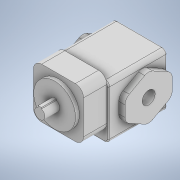
# Autodesk Inventor part: Motor Pump
Saved by Autodesk Inventor 2020 (Build 240168000, 168)
## iProperties
Created: 2020-10-14
Part Number: Motor Pump
Material: Generic
Document SubType Name: Modeling
Designer: jtri402
Density: 1 g/cm^3
Appearance: Default
Author: jtri402
Autodesk Inventor part; units mm, degrees
ref_plane "YZ Plane" through (0, 0, 0) normal (1, 0, 0) x (0, 1, 0)
sketch "Sketch1" plane through (0, 0, 0) normal (0, 0, 1) x (1, 0, 0)
  line L0 (-65, 65) -> (65, 65)
  line L1 (65, 65) -> (65, -65)
  line L2 (65, -65) -> (-65, -65)
  line L3 (-65, -65) -> (-65, 65)
  point P0 (0, 0)
  dimension "d0" = 130
  dimension "d1" = 130
  dimension "d2" = 65
  dimension "d3" = 65
  constraints: 8 end point, 2 parallel, 1 horizontal, 1 perpendicular
  measures "d0" distance of L0.start L0.end
  measures "d1" distance of L0.end L1.end
  measures "d2" distance from line of point (0, 0) L0
  measures "d3" distance from line of L1 point (0, 0)
extrude "Extrusion1" add sketch "Sketch1" along normal blind 203.2
ref_plane "Work Plane2" through (65, -55, 2) normal (1, 0, 0) x (0, 0, -1)
sketch "Sketch2" plane through (65, -55, 2) normal (1, 0, 0) x (0, 0, -1)
  line L0 (0, 110) -> (0, 0) projected
  line L1 (-115, 80) -> (0, 80)
  line L2 (0, 80) -> (0, 30)
  line L3 (0, 30) -> (-115, 30)
  line L4 (-115, 30) -> (-115, 80)
  line L5 (-201.2, -10) -> (2, -10) projected
  line L6 (2, 120) -> (-201.2, 120) projected
  line L7 (-57.5, 111.6) -> (-115, 80)
  line L8 (-57.5, 111.6) -> (0, 80)
  line L9 (-57.5, -1.6) -> (-115, 30)
  line L10 (-57.5, -1.6) -> (0, 30)
  point P0 (2, 55)
  point P1 (-199.2, -10)
  point P2 (0, -10)
  point P3 (0, 120)
  point P4 (-199.2, 120)
  point P5 (0, 80)
  dimension "d8" = 50
  dimension "d9" = 115
  dimension "d10" = 130
  dimension "d11" = 40
  constraints: 16 end point, 4 parallel, 1 horizontal, 1 perpendicular, 1 point on line
  measures "d8" distance of L3.end L1.start
  measures "d9" distance of L1.start L1.end
  measures "d10" distance between parallel lines of L5 L6
  measures "d11" distance between parallel lines of L1 L6
extrude "Extrusion2" add sketch "Sketch2" along normal blind 15
sketch "Sketch3" plane through (80, -55, 2) normal (1, 0, 0) x (0, 0, -1)
  circle A0 centre (-57.5, 55) radius 15.8
  point P0 (2, 55)
  dimension "d18" = 31.6
  constraints: 1 centre point
  measures "d18" diameter of A0
ref_plane "Work Plane1" through (-65, -55, 2) normal (-1, 0, 0) x (0, 0, 1)
sketch "Sketch4" plane through (-65, -55, 2) normal (-1, 0, 0) x (0, 0, 1)
  line L0 (0, 110) -> (0, 68.1701) projected
  line L1 (0, 80) -> (115.3, 80)
  line L2 (115.3, 80) -> (115.3, 30)
  line L3 (115.3, 30) -> (0, 30)
  line L4 (0, 30) -> (0, 80)
  line L5 (201.2, 120) -> (-2, 120) projected
  line L6 (-2, -10) -> (201.2, -10) projected
  line L7 (0, 80) -> (57.5, 110.755)
  arc A0 (60.3849, 110.0145) -> (54.6151, 110.0145) centre (57.5, 104.765) ccw projected
  line L8 (60.3849, 110.0145) -> (104.6325, 85.6976) projected
  line L9 (57.5, 110.755) -> (115.3, 80)
  line L10 (115.3, 30) -> (57.8, -0.755)
  line L11 (57.8, -0.755) -> (0, 30)
  point P0 (-2, 55)
  point P1 (199.2, 120)
  point P2 (0, 120)
  point P3 (0, -10)
  point P4 (199.2, -10)
  dimension "d19" = 115.3
  dimension "d20" = 50
  dimension "d21" = 40
  dimension "d22" = 130
  constraints: 16 end point, 4 parallel, 1 horizontal, 1 perpendicular, 1 point on circle, 1 point on line
  measures "d19" distance of L1.start L1.end
  measures "d20" distance of L3.end L1.start
  measures "d21" distance between parallel lines of L1 L5
  measures "d22" distance between parallel lines of L6 L5
extrude "Extrusion3" add sketch "Sketch4" along normal blind 15
extrude "Extrusion4" cut sketch "Sketch3" against normal blind 160
sketch "Sketch6" plane through (0, 0, 203.2) normal (0, 0, 1) x (1, 0, 0)
  line L0 (-65, 65) -> (-65, -65) projected
  line L1 (65, -65) -> (65, 65) projected
  line L2 (-65, 65) -> (65, 65)
  line L3 (65, 65) -> (65, -65)
  line L4 (65, -65) -> (-65, -65)
  line L5 (-65, -65) -> (-65, 65)
  point P0 (0, 0)
  constraints: 8 end point, 2 parallel, 1 horizontal, 1 perpendicular
extrude "Extrusion5" cut sketch "Sketch6" against normal blind 60.9
fillet "Fillet8" radius 3 8 edges at (0, 65, 142.3) (65, 0, 142.3) (0, -65, 142.3) (-65, 0, 142.3) (65, 0, 0) (0, 65, 0) (-65, 0, 0) (0, -65, 0)
fillet "Fillet8" radius 10 4 edges at (65, 65, 71.15) (-65, 65, 71.15) (-65, -65, 71.15) (65, -65, 71.15)
fillet "Fillet8" radius 20 12 edges at (72.5, 56.6, 59.5) (72.5, 25, 117) (72.5, -25, 117) (72.5, -25, 2) (72.5, 25, 2) (72.5, -56.6, 59.5) (-72.5, -55.755, 59.8) (-72.5, -25, 2) (-72.5, 25, 2) (-72.5, 55.755, 59.5) (-72.5, 25, 117.3) (-72.5, -25, 117.3)
sketch "Sketch7" plane through (0, 0, 142.3) normal (0, 0, 1) x (1, 0, 0)
  line L0 (-61, 79.5) -> (61, 79.5)
  line L1 (61, 79.5) -> (61, -42.5)
  line L2 (61, -42.5) -> (-61, -42.5)
  line L3 (-61, -42.5) -> (-61, 79.5)
  line L4 (-65, 55) -> (-65, -55) projected
  line L5 (-55, -65) -> (55, -65) projected
  point P0 (0, 0)
  dimension "d38" = 122
  dimension "d39" = 122
  dimension "d40" = 4
  dimension "d41" = 22.5
  constraints: 8 end point, 2 parallel, 1 horizontal, 1 perpendicular
  measures "d38" distance of L0.start L0.end
  measures "d39" distance of L0.end L1.end
  measures "d40" distance between parallel lines of L3 L4
  measures "d41" distance between parallel lines of L5 L2
extrude "Extrusion6" add sketch "Sketch7" along normal blind 56.5
fillet "Fillet9" radius 20 4 edges at (-61, 79.5, 170.55) (-61, -42.5, 170.55) (61, 79.5, 170.55) (61, -42.5, 170.55)
sketch "Sketch8" plane through (0, 0, 198.8) normal (0, 0, 1) x (1, 0, 0)
  circle A0 centre (0, 18.5) radius 50.8
  line L0 (41, 79.5) -> (-41, 79.5) projected
  point P0 (0, 0)
  dimension "d45" = 101.6
  dimension "d46" = 61
  constraints: 1 centre point
  measures "d45" diameter of A0
  measures "d46" distance from line of A0.centre L0
extrude "Extrusion7" add sketch "Sketch8" along normal blind 9.4
sketch "Sketch9" plane through (0, 18.5, 208.2) normal (0, 0, 1) x (1, 0, 0)
  circle A0 centre (0, 0) radius 12.5
  point P0 (0, -18.5)
  dimension "d49" = 25
  constraints: 1 centre point
  measures "d49" diameter of A0
extrude "Extrusion8" add sketch "Sketch9" along normal blind 36.1
sketch "Sketch10" plane through (0, 18.5, 244.3) normal (0, 0, 1) x (1, 0, 0)
  line L0 (-4, 15) -> (4, 15)
  line L1 (4, 15) -> (4, 10)
  line L2 (4, 10) -> (-4, 10)
  line L3 (-4, 10) -> (-4, 15)
  circle A0 centre (0, 0) radius 12.5 projected
  point P0 (0, -18.5)
  point P1 (-4, 11.8427)
  point P2 (4, 11.8427)
  dimension "d52" = 8
  dimension "d53" = 5
  dimension "d54" = 2.5
  dimension "d55" = 4
  constraints: 8 end point, 2 parallel, 1 horizontal, 1 perpendicular
  measures "d52" distance of L1.end L2.end
  measures "d53" distance of L2.end L0.start
  measures "d54" distance edge to line of A0 L2
  measures "d55" distance from line of A0.centre L1
extrude "Extrusion9" add sketch "Sketch10" against normal blind 36.1 contours L0 L1 A0 L3
body "Solid1"
